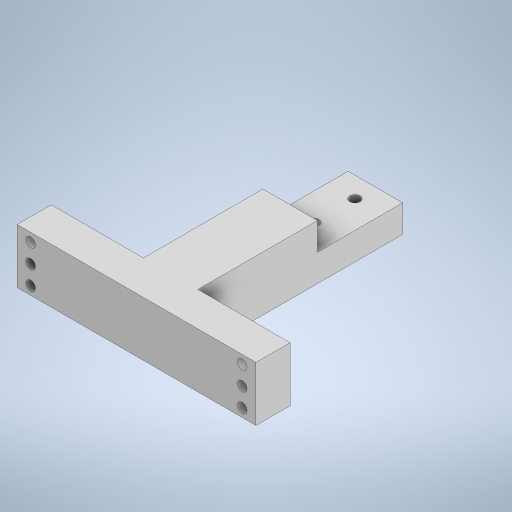
# Autodesk Inventor part: B1_head_T
Saved by Autodesk Inventor 2023.1 (Build 271208000, 208)
## iProperties
Created: 2023-06-14
Part Number: B1_head_T
Material: Generic
Document SubType Name: Modeling
Designer: zavrel
Density: 1 g/cm^3
Appearance: Default
Author: zavrel
Autodesk Inventor part; units mm, degrees
ref_plane "YZ Plane" through (0, 0, 0) normal (1, 0, 0) x (0, 1, 0)
ref_plane "XZ Plane" through (0, 0, 0) normal (0, 1, 0) x (-1, 0, 0)
ref_plane "XY Plane" through (0, 0, 0) normal (0, 0, 1) x (1, 0, 0)
sketch "Sketch1" plane through (0, 0, 0) normal (0, 1, 0) x (-1, 0, 0)
  line L0 (0, -29.3233) -> (8, -29.3233)
  line L1 (8, -29.3233) -> (8, 30.6767)
  line L2 (0, 0) -> (0, -29.3233) construction
  line L3 (0, -29.3233) -> (-8, -29.3233)
  line L4 (-8, -29.3233) -> (-8, 30.6767)
  line L5 (8, 30.6767) -> (35, 30.6767)
  line L6 (35, 30.6767) -> (35, 40.6767)
  line L7 (35, 40.6767) -> (2.1646, 40.6767)
  line L8 (2.1646, 40.6767) -> (0, 40.6767)
  line L9 (-8, 30.6767) -> (-35, 30.6767)
  line L10 (-35, 30.6767) -> (-35, 40.6767)
  line L11 (-35, 40.6767) -> (-2.1646, 40.6767)
  line L12 (-2.1646, 40.6767) -> (0, 40.6767)
  point P0 (4, -29.3233)
  point P1 (-4, -29.3233)
  dimension "d0" = 16
  dimension "d17" = 10
  dimension "d32" = 70
  dimension "d35" = 70
  constraints: 26 end point, 5 symmetric about line, 4 perpendicular, 2 midpoint, 1 collinear, 1 horizontal, 1 point on line, 1 vertical
  measures "d0" distance between parallel lines of L4 L1
  measures "d17" distance between parallel lines of L7 L5
  measures "d32" distance from line of point (-4, -29.323) L11
  measures "d35" distance between parallel lines of L10 L6
extrude "Extrusion1" add sketch "Sketch1" along normal blind 16
sketch "Sketch2" plane through (0, 16, 0) normal (0, 1, 0) x (1, 0, 0)
  line L0 (8, 29.3233) -> (-8, 29.3233) projected
  line L1 (-8, 29.3233) -> (-8, -30.6767) projected
  line L2 (8, -30.6767) -> (8, 29.3233) projected
  line L3 (8, -30.6767) -> (8, 29.3233) projected
  line L4 (-8, 29.3233) -> (8, 29.3233)
  line L5 (8, 29.3233) -> (8, 4.3233)
  line L6 (8, 4.3233) -> (-8, 4.3233)
  line L7 (-8, 4.3233) -> (-8, 29.3233)
  line L8 (-8, -30.6767) -> (-35, -30.6767) projected
  line L9 (-35, -30.6767) -> (-35, -40.6767) projected
  line L10 (-35, -40.6767) -> (35, -40.6767) projected
  line L11 (35, -40.6767) -> (35, -30.6767) projected
  line L12 (35, -30.6767) -> (8, -30.6767) projected
  point P0 (0, 0)
  point P1 (-8, 4.3233)
  dimension "d6" = 25
  constraints: 8 end point, 2 parallel, 1 horizontal, 1 perpendicular, 1 point on line
  measures "d6" distance between parallel lines of L0 L6
extrude "Extrusion2" cut sketch "Sketch2" against normal blind 8 contours L2 L6 L1 L0
sketch "Sketch3" plane through (0, 0, 0) normal (0, -1, 0) x (1, 0, 0)
  line L0 (8, -29.3233) -> (-8, -29.3233) projected
  line L1 (8, 30.6767) -> (8, -29.3233) projected
  line L2 (-8, -29.3233) -> (-8, 30.6767) projected
  circle A0 centre (0, -23.3233) radius 1.5
  circle A1 centre (0, -11.3233) radius 1.5
  line L3 (35, 30.6767) -> (8, 30.6767) projected
  line L4 (35, 40.6767) -> (35, 30.6767) projected
  line L5 (-35, 40.6767) -> (35, 40.6767) projected
  line L6 (-35, 30.6767) -> (-35, 40.6767) projected
  line L7 (-8, 30.6767) -> (-35, 30.6767) projected
  point P0 (0, 0)
  dimension "d9" = 3
  dimension "d10" = 6
  dimension "d11" = 12
  constraints: 2 centre point, 1 equal radius
  measures "d9" diameter of A0
  measures "d10" distance from line of A0.centre L0
  measures "d11" distance of A0.centre A1.centre
extrude "Extrusion3" cut sketch "Sketch3" against normal through all contours A0 | A1
sketch "Sketch4" plane through (0, 0, 0) normal (0, -1, 0) x (1, 0, 0)
  circle A0 centre (0, -11.3233) radius 1.5 projected
  circle A1 centre (0, -23.3233) radius 1.5 projected
  line L0 (8, -29.3233) -> (-8, -29.3233) projected
  line L1 (8, 30.6767) -> (8, -29.3233) projected
  line L2 (-8, -29.3233) -> (-8, 30.6767) projected
  circle A2 centre (0, -23.3233) radius 3
  circle A3 centre (0, -11.3233) radius 1.5 projected
  circle A4 centre (0, -11.3233) radius 3
  line L3 (35, 30.6767) -> (8, 30.6767) projected
  line L4 (35, 40.6767) -> (35, 30.6767) projected
  line L5 (-35, 40.6767) -> (35, 40.6767) projected
  line L6 (-35, 30.6767) -> (-35, 40.6767) projected
  line L7 (-8, 30.6767) -> (-35, 30.6767) projected
  point P0 (0, 0)
  dimension "d14" = 6
  constraints: 2 centre point, 2 coincident, 1 equal radius
  measures "d14" diameter of A4
extrude "Extrusion4" cut sketch "Sketch4" against normal blind 3 contours A2 | A4
sketch "Sketch5" plane through (0.8354, 0, 40.6767) normal (0, 0, 1) x (1, 0, 0)
  line L0 (-35.8354, 0) -> (34.1646, 0) projected
  line L1 (-35.8354, 16) -> (34.1646, 16) projected
  line L2 (-35.8354, 0) -> (-35.8354, 16) projected
  line L3 (-35.8354, 0) -> (-35.8354, 16) construction
  line L4 (-35.8354, 8) -> (34.1646, 8) construction
  circle A0 centre (-31.8354, 13.5) radius 1.4
  circle A1 centre (-31.8354, 8) radius 1.4
  circle A2 centre (-31.8354, 2.5) radius 1.4
  line L5 (34.1646, 0) -> (34.1646, 16) projected
  line L6 (-35.8354, 16) -> (34.1646, 16) construction
  line L7 (-0.8354, 16) -> (-0.8354, 0) construction
  line L8 (-35.8354, 0) -> (34.1646, 0) projected
  circle A3 centre (30.1646, 13.5) radius 1.4
  circle A4 centre (30.1646, 8) radius 1.4
  circle A5 centre (30.1646, 2.5) radius 1.4
  dimension "d19" = 2.8
  dimension "d20" = 11
  dimension "d21" = 4
  constraints: 6 centre point, 4 end point, 4 midpoint, 4 symmetric about line, 1 equal radius, 1 point on line, 1 vertical alignment, 4 other
  measures "d19" diameter of A0
  measures "d20" distance of A2.centre A0.centre
  measures "d21" distance from line of L2 A1.centre
extrude "Extrusion8" cut sketch "Sketch5" against normal through all contours A0 | A1 | A2 | A3 | A4 | A5
body "Solid1"
